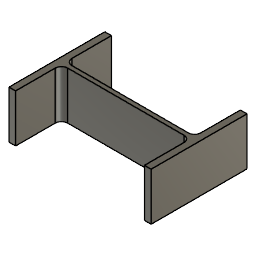
H-298×201×9×14 (Autodesk Fusion 360 design; units mm, degrees)
Autodesk Fusion 360 part; units mm, degrees
sketch "スケッチ1" plane through (0, 0, 0) normal (0, 0, 1) x (1, 0, 0)
  line L0 (0, 100.5) -> (0, -100.5)
  line L1 (14, 17.5) -> (14, 100.5)
  line L2 (284, 100.5) -> (284, 17.5)
  line L3 (298, -100.5) -> (298, 100.5)
  line L4 (284, -17.5) -> (284, -100.5)
  line L5 (14, -100.5) -> (14, -17.5)
  line L6 (0, -100.5) -> (14, -100.5)
  line L7 (284, -100.5) -> (298, -100.5)
  line L8 (271, 4.5) -> (27, 4.5)
  line L9 (27, -4.5) -> (271, -4.5)
  line L10 (14, 100.5) -> (0, 100.5)
  line L11 (298, 100.5) -> (284, 100.5)
  arc A0 (27, -4.5) -> (14, -17.5) centre (27, -17.5) ccw
  arc A1 (14, 17.5) -> (27, 4.5) centre (27, 17.5) ccw
  arc A2 (271, 4.5) -> (284, 17.5) centre (271, 17.5) ccw
  arc A3 (284, -17.5) -> (271, -4.5) centre (271, -17.5) ccw
extrude "押し出し1" add sketch "スケッチ1" along normal blind 100
